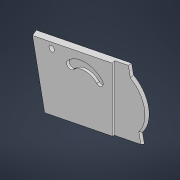
# Autodesk Inventor part: Deo1 with Sketch
Saved by Autodesk Inventor 2022.1 (Build 261234000, 234)
## iProperties
Created: 2021-08-16
Part Number: Deo1 with Sketch
Material: Generic
Document SubType Name: Modeling
Designer: Nedeljko Š.
Density: 1 g/cm^3
Appearance: Default
Author: Nedeljko Š.
Autodesk Inventor part; units mm, degrees
ref_plane "YZ Plane" through (0, 0, 0) normal (1, 0, 0) x (0, 1, 0)
ref_plane "XZ Plane" through (0, 0, 0) normal (0, 1, 0) x (-1, 0, 0)
ref_plane "XY Plane" through (0, 0, 0) normal (0, 0, 1) x (1, 0, 0)
sketch "Sketch1" plane through (0, 0, 0) normal (0, 0, 1) x (1, 0, 0)
  line L0 (-76.521, -76.4496) -> (100, -41.2311)
  line L1 (100, -41.2311) -> (76.521, 76.4496)
  line L2 (76.521, 76.4496) -> (-100, 41.2311)
  line L3 (-100, 41.2311) -> (-76.521, -76.4496)
  line L4 (-76.521, -76.4496) -> (76.521, 76.4496) construction
  line L5 (100, -41.2311) -> (-100, 41.2311) construction
  point P0 (0, 0)
  point P1 (0, 0)
  dimension "d0" = 180
  dimension "d1" = 120
  dimension "d23" = 100
  constraints: 12 end point, 3 midpoint, 2 parallel, 1 perpendicular
  measures "d0" distance of L2.end L1.end
  measures "d1" distance of L1.end L0.end
  measures "d23" horizontal distance of point (0, 0) L2.end
extrude "Extrusion1" add sketch "Sketch1" along normal blind 10 draft -15
sketch "Sketch2" plane through (0, 0, 0) normal (0, 0, 1) x (1, 0, 0)
  circle A0 centre (53.937, 10.7612) radius 55
  line L0 (100, -41.2311) -> (76.521, 76.4496) construction
  line L1 (0, 0) -> (88.2605, 17.6093) construction
  dimension "d1" = 120
  dimension "d4" = 110
  dimension "d5" = 55
  constraints: 2 end point, 1 centre point, 1 midpoint, 1 point on line
  measures "d4" diameter of A0
  measures "d5" distance of A0.centre L1.start
extrude "Extrusion2" add sketch "Sketch2" along normal blind 10 draft -30
sketch "Sketch3" plane through (0, 0, 10) normal (0, 0, 1) x (1, 0, 0)
  line L0 (-74.4175, -73.2976) -> (-96.848, 39.1276) projected
  line L1 (-96.848, 39.1276) -> (74.4175, 73.2976) projected
  point P0 (0, 0)
  point P1 (-61.4584, 35.8123)
hole "Hole1" at (-61.4584, 35.8123, 10) direction (0, 0, -1) diameter 10 depth 18
sketch "Sketch4" plane through (0, 0, 10) normal (0, 0, 1) x (1, 0, 0)
  arc A0 (26.8701, 26.8701) -> (-26.8701, 26.8701) centre (0, 0) ccw construction
  arc A1 (31.8198, 31.8198) -> (-31.8198, 31.8198) centre (0, 0) ccw
  arc A2 (21.9203, 21.9203) -> (-21.9203, 21.9203) centre (0, 0) ccw
  arc A3 (21.9203, 21.9203) -> (31.8198, 31.8198) centre (26.8701, 26.8701) ccw
  arc A4 (-31.8198, 31.8198) -> (-21.9203, 21.9203) centre (-26.8701, 26.8701) ccw
  dimension "d18" = 90
  dimension "d19" = 7
  dimension "d20" = 38
  constraints: 10 point on circle, 5 centre point, 4 tangent, 1 coincident, 1 horizontal alignment
  measures "d19" radius of A3
  measures "d20" radius of A0
extrude "Extrusion3" cut sketch "Sketch4" against normal blind 5
sketch "Sketch6" plane through (0, 0, 10) normal (0, 0, 1) x (1, 0, 0)
  line L0 (50.4655, 83.5966) -> (130.9866, 83.5966)
  line L1 (130.9866, 83.5966) -> (130.9866, -61.5092)
  line L2 (130.9866, -61.5092) -> (50.4655, -61.5092)
  line L3 (50.4655, -61.5092) -> (50.4655, 83.5966)
  point P0 (0, 0)
  dimension "d1" = 120
  constraints: 8 end point, 2 parallel, 1 horizontal, 1 perpendicular
extrude "Extrusion4" cut sketch "Sketch6" against normal up to surface (5 mm away)
body "Solid1"
